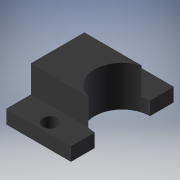
# Autodesk Inventor part: UCover_SMA
Saved by Autodesk Inventor 2019.4 (Build 234330000, 330)
## iProperties
Created: 2020-06-11
Part Number: UCover_SMA
Material: Generic
Document SubType Name: Modeling
Designer: ions
Density: 1 g/cm^3
Appearance: Default
Author: ions
Autodesk Inventor part; units mm, degrees
ref_plane "YZ Plane" through (0, 0, 0) normal (1, 0, 0) x (0, 1, 0)
ref_plane "XZ Plane" through (0, 0, 0) normal (0, 1, 0) x (-1, 0, 0)
ref_plane "XY Plane" through (0, 0, 0) normal (0, 0, 1) x (1, 0, 0)
sketch "Sketch1" plane through (0, 0, 0) normal (0, 1, 0) x (-1, 0, 0)
  line L0 (1.7184, 7.0425) -> (-7.8416, 7.0425)
  line L1 (-7.8416, -8.1575) -> (1.7184, -8.1575)
  line L2 (1.7184, -8.1575) -> (1.7184, 7.0425)
  circle A0 centre (-3.2816, 5.5425) radius 1.15
  circle A1 centre (-3.2816, -6.6575) radius 1.15
  line L3 (-7.8416, 7.0425) -> (-7.8416, 3.5425)
  line L4 (-7.8416, -4.6575) -> (-7.8416, -8.1575)
  arc A2 (-7.8416, -4.6575) -> (-7.8416, 3.5425) centre (-7.8416, -0.5575) ccw
  point P0 (0, 0)
  dimension "d0" = 15.2
  dimension "d2" = 5
  dimension "d3" = 5
  dimension "d4" = 1.5
  dimension "d5" = 1.5
  dimension "d6" = 2.3
  dimension "d7" = 2.3
  dimension "d11" = 9.56
  dimension "d12" = 8.2
  dimension "d13" = 7.6
  constraints: 10 end point, 3 centre point, 3 parallel, 2 perpendicular, 2 point on circle, 1 horizontal
  measures "d0" distance between parallel lines of L1 L0
  measures "d2" distance from line of A0.centre L2
  measures "d3" distance from line of A1.centre L2
  measures "d4" distance from line of L0 A0.centre
  measures "d5" distance from line of L1 A1.centre
  measures "d6" diameter of A0
  measures "d7" diameter of A1
  measures "d11" distance between parallel lines of L3 L2
  measures "d12" diameter of A2
  measures "d13" distance from line of A2.centre L0
extrude "Extrusion1" add sketch "Sketch1" along normal blind 6
sketch "Sketch2" plane through (0, 6, 0) normal (0, 1, 0) x (1, 0, 0)
  line L0 (-1.7184, -7.0425) -> (7.8416, -7.0425) projected
  line L1 (-1.7184, 8.1575) -> (-1.7184, -7.0425) projected
  line L2 (7.8416, -7.0425) -> (-1.7184, -7.0425)
  line L3 (-1.7184, -7.0425) -> (-1.7184, -3.3925)
  line L4 (-1.7184, -3.3925) -> (7.8416, -3.3925)
  line L5 (7.8416, -3.3925) -> (7.8416, -7.0425)
  line L6 (7.8416, 4.5075) -> (-1.7184, 4.5075)
  line L7 (-1.7184, 4.5075) -> (-1.7184, 8.1575)
  line L8 (-1.7184, 8.1575) -> (7.8416, 8.1575)
  line L9 (7.8416, 8.1575) -> (7.8416, 4.5075)
  point P0 (0, 0)
  dimension "d14" = 3.65
  dimension "d19" = 3.65
  constraints: 16 end point, 4 parallel, 2 horizontal, 2 perpendicular, 2 point on line
  measures "d14" distance between parallel lines of L0 L4
  measures "d19" distance of L8.end L6.start
extrude "Extrusion2" cut sketch "Sketch2" against normal blind 4 contours L1 L4 L5 L0
extrude "Extrusion3" cut sketch "Sketch2" against normal blind 4 contours L1 L8 L9 L6
body "Solid1"
